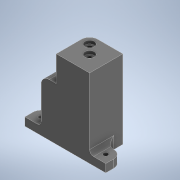
# Autodesk Inventor part: IdlerBlock10mm
Saved by Autodesk Inventor 2022 (Build 260153000, 153)
## iProperties
Created: 2021-06-16
Part Number: IdlerBlock10mm
Material: Generic
Document SubType Name: Modeling
Designer: burgessb
Density: 1 g/cm^3
Appearance: Gray
Author: burgessb
Autodesk Inventor part; units mm, degrees
ref_plane "YZ Plane" through (0, 0, 0) normal (1, 0, 0) x (0, 1, 0)
ref_plane "XZ Plane" through (0, 0, 0) normal (0, 1, 0) x (-1, 0, 0)
ref_plane "XY Plane" through (0, 0, 0) normal (0, 0, 1) x (1, 0, 0)
sketch "Sketch1" plane through (0, 0, 0) normal (0, 1, 0) x (-1, 0, 0)
  circle A0 centre (0, 0) radius 3.25
  circle A1 centre (0, 0) radius 10
  circle A2 centre (11.1, -11.1) radius 3.25
  circle A3 centre (11.1, -11.1) radius 10
  line L0 (-10, 0) -> (-10, -21.1)
  line L1 (-10, -21.1) -> (11.1, -21.1)
  line L2 (0, 10) -> (21.1, 10)
  line L3 (21.1, 10) -> (21.1, -11.1)
  line L4 (-10, -21.1) -> (-20, -21.1)
  line L5 (-20, -21.1) -> (-20, 20)
  line L6 (-20, 20) -> (-10, 20)
  line L7 (-10, 20) -> (-10, -21.1)
  line L8 (21.1, 10) -> (-10, 10)
  line L9 (-10, 10) -> (-10, 20)
  line L10 (-10, 20) -> (21.1, 20)
  line L11 (21.1, 20) -> (21.1, 10)
  circle A4 centre (0, 0) radius 7.5
  circle A5 centre (11.1, -11.1) radius 7.5
  point P0 (1.1685, -9.9315)
  point P1 (9.9315, -1.1685)
  dimension "d0" = 6.5
  dimension "d1" = 20
  dimension "d2" = 6.5
  dimension "d3" = 20
  dimension "d4" = 11.1
  dimension "d5" = 11.1
  dimension "d8" = 10
  dimension "d9" = 10
  dimension "d10" = 15
  dimension "d11" = 15
  constraints: 24 end point, 6 centre point, 5 coincident, 4 parallel, 4 perpendicular, 4 point on circle, 4 tangent, 3 horizontal, 1 vertical
  measures "d0" diameter of A0
  measures "d1" diameter of A1
  measures "d2" diameter of A2
  measures "d3" diameter of A3
  measures "d4" horizontal distance of A2.centre point (0, 0)
  measures "d5" horizontal distance of A2.centre point (0, 0)
  measures "d8" distance of L5.end L6.end
  measures "d9" distance of L10.end L2.end
  measures "d10" diameter of A4
  measures "d11" diameter of A5
extrude "Extrusion1" add sketch "Sketch1" along normal blind 10
sketch "Sketch2" plane through (0, 0, 0) normal (0, -1, 0) x (1, 0, 0)
  circle A0 centre (-11.1, -11.1) radius 3.25 projected
  circle A1 centre (0, 0) radius 3.25 projected
  line L0 (-21.1, 20) -> (20, 20) projected
  line L1 (-21.1, -11.1) -> (-21.1, 20) projected
  arc A2 (-21.1, -11.1) -> (-11.1, -21.1) centre (-11.1, -11.1) ccw projected
  line L2 (20, -21.1) -> (-11.1, -21.1) projected
  line L3 (20, 20) -> (20, -21.1) projected
  circle A3 centre (0, 0) radius 10
  line L4 (0, 10) -> (-21.1, 10)
  line L5 (-21.1, -11.1) -> (-21.1, 20) projected
  line L6 (10, 0) -> (10, -21.1)
  line L7 (20, -21.1) -> (-11.1, -21.1) projected
  dimension "d12" = 20
  constraints: 4 end point, 2 perpendicular, 2 point on circle, 2 point on line, 2 tangent, 1 centre point, 1 coincident
  measures "d12" diameter of A3
extrude "Extrusion2" add sketch "Sketch2" along normal blind 22 contours L0 L3 L2 L6 A3 L4 L1
sketch "Sketch3" plane through (0, -22, 0) normal (0, -1, 0) x (1, 0, 0)
  line L0 (-21.1, 20) -> (20, 20) projected
  line L1 (20, 20) -> (-40, 20)
  line L2 (-40, 20) -> (-40, -21.1)
  line L3 (-40, -21.1) -> (20, -21.1)
  line L4 (20, -21.1) -> (20, 20)
  circle A0 centre (-11.1, -11.1) radius 3.25 projected
  circle A1 centre (0, 0) radius 3.25 projected
  dimension "d15" = 60
  dimension "d16" = 41.1
  constraints: 8 end point, 2 parallel, 1 horizontal, 1 perpendicular
  measures "d15" distance of L3.end L2.end
  measures "d16" distance of L2.end L1.end
extrude "Extrusion3" add sketch "Sketch3" along normal blind 65
sketch "Sketch4" plane through (20, 10, -21.1) normal (0, 0, -1) x (-1, 0, 0)
  circle A0 centre (51, -43) radius 5.25
  line L0 (60, -32) -> (10, -32) projected
  line L1 (60, -32) -> (60, -97) projected
  point P0 (20, -10)
  dimension "d19" = 10.5
  dimension "d20" = 11
  dimension "d21" = 9
  constraints: 1 centre point
  measures "d19" diameter of A0
  measures "d20" distance from line of L0 A0.centre
  measures "d21" distance from line of L1 A0.centre
extrude "Extrusion4" cut sketch "Sketch4" against normal blind 30
fillet "Fillet1" radius 10 1 edges at (-40, -22, -0.55)
sketch "Sketch5" plane through (0, 10, 0) normal (0, 1, 0) x (1, 0, 0)
  circle A0 centre (-11.1, 11.1) radius 3.25 projected
  circle A1 centre (0, 0) radius 3.25 projected
  line L0 (-21.1, -20) -> (20, -20) projected
  line L1 (20, -20) -> (20, 21.1) projected
  line L2 (20, 21.1) -> (-11.1, 21.1) projected
  arc A2 (-11.1, 21.1) -> (-21.1, 11.1) centre (-11.1, 11.1) ccw projected
  line L3 (-21.1, 11.1) -> (-21.1, -20) projected
  circle A3 centre (0, 0) radius 5.75
  circle A4 centre (-11.1, 11.1) radius 5.75
  dimension "d25" = 11.5
  dimension "d26" = 11.5
  constraints: 2 centre point, 2 coincident
  measures "d25" diameter of A3
  measures "d26" diameter of A4
extrude "Extrusion5" cut sketch "Sketch5" against normal blind 4 contours A3 | A4
sketch "Sketch6" plane through (0, -87, 0) normal (0, -1, 0) x (1, 0, 0)
  circle A0 centre (0, 0) radius 5.75 projected
  circle A1 centre (-11.1, -11.1) radius 5.75 projected
extrude "Extrusion6" cut sketch "Sketch6" against normal blind 54
sketch "Sketch7" plane through (0, -87, 0) normal (0, -1, 0) x (1, 0, 0)
  circle A0 centre (-11.1, -11.1) radius 5.75 projected
  circle A1 centre (0, 0) radius 5.75 projected
  line L0 (20, 20) -> (-40, 20) projected
  line L1 (-40, 20) -> (-40, -21.1) projected
  line L2 (-40, -21.1) -> (20, -21.1) projected
  line L3 (20, -21.1) -> (20, 20) projected
  circle A2 centre (30, 10) radius 2.75
  circle A3 centre (-50, 10) radius 2.75
  circle A4 centre (-10, -31.1) radius 2.75
  circle A5 centre (30, 10) radius 10
  circle A6 centre (-50, 10) radius 10
  line L4 (20, 20) -> (40, 20)
  line L5 (40, 20) -> (40, 10)
  line L6 (30, 0) -> (20, 0)
  line L7 (20, 20) -> (20, -21.1) projected
  line L8 (-50, 0) -> (-40, 0)
  line L9 (-40, -21.1) -> (-40, 20) projected
  line L10 (-60, 10) -> (-60, 20)
  line L11 (-60, 20) -> (-40, 20)
  circle A7 centre (-10, -31.1) radius 10
  line L12 (0, -31.1) -> (0, -21.1)
  line L13 (-30, -21.1) -> (10, -21.1) projected
  line L14 (-20, -31.1) -> (-20, -21.1)
  dimension "d31" = 5.5
  dimension "d32" = 5.5
  dimension "d33" = 5.5
  dimension "d34" = 60
  dimension "d35" = 30
  dimension "d36" = 10
  dimension "d37" = 10
  dimension "d38" = 20
  dimension "d39" = 20
  dimension "d40" = 10
  dimension "d41" = 10
  dimension "d42" = 20
  dimension "d43" = 10
  constraints: 16 end point, 6 centre point, 6 point on circle, 6 point on line, 5 tangent, 4 perpendicular, 3 coincident, 1 horizontal, 1 vertical
  measures "d31" diameter of A2
  measures "d32" diameter of A3
  measures "d33" diameter of A4
  measures "d34" distance of L0.start L0.end
  measures "d35" horizontal distance of L1.end A4.centre
  measures "d36" distance from line of L0 A3.centre
  measures "d37" distance from line of L0 A2.centre
  measures "d38" diameter of A5
  measures "d39" diameter of A6
  measures "d40" distance from line of L3 A2.centre
  measures "d41" distance from line of L1 A3.centre
  measures "d42" diameter of A7
  measures "d43" distance from line of L2 A7.centre
extrude "Extrusion7" add sketch "Sketch7" against normal blind 10 contours L4 A5 L3 | L1 A6 L11 | A5 L6 L3 | A5 | L4 L5 A5 | L1 L8 A6 | A6 | A6 L10 L11 | L12 A7 L2 | L2 A7 L14 | A7
fillet "Fillet2" radius 10 4 edges at (20, -82, 0) (0, -82, -21.1) (-20, -82, -21.1) (-40, -82, 0)
fillet "Fillet3" radius 5 3 edges at (20, -77, 10) (-10, -77, -21.1) (-40, -77, 10)
equation "\"d3\" = d1"
equation "\"d5\" = d4"
equation "\"d9\" = d8"
equation "\"d35\" = 0.5 * d34"
equation "\"d43\" = 0.5 * d42"
equation "\"d44\" = d41"
body "Solid1"
